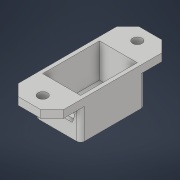
# Autodesk Inventor part: Caixa mlx
Saved by Autodesk Inventor 2021 (Build 250183000, 183)
## iProperties
Created: 2022-03-10
Part Number: Caixa mlx
Material: Genérico
Document SubType Name: Modeling
Designer: Hanter
Density: 1 g/cm^3
Appearance: Padrão
Author: Hanter
Autodesk Inventor part; units mm, degrees
ref_plane "YZ Plane" through (0, 0, 0) normal (1, 0, 0) x (0, 1, 0)
ref_plane "XZ Plane" through (0, 0, 0) normal (0, 1, 0) x (-1, 0, 0)
ref_plane "XY Plane" through (0, 0, 0) normal (0, 0, 1) x (1, 0, 0)
sketch "Esboço1" plane through (0, 0, 0) normal (0, 1, 0) x (-1, 0, 0)
  line L0 (-12, 17) -> (12, 17)
  line L1 (12, 17) -> (12, -17)
  line L2 (12, -17) -> (-12, -17)
  line L3 (-12, -17) -> (-12, 17)
  line L4 (-12, 17) -> (12, -17) construction
  line L5 (12, 17) -> (-12, -17) construction
  point P0 (0, 0)
  dimension "d0" = 24
  dimension "d1" = 34
  constraints: 12 end point, 2 midpoint, 2 parallel, 1 horizontal, 1 perpendicular
  measures "d0" distance of L1.end L2.end
  measures "d1" distance of L0.end L1.end
extrude "Extrusão1" add sketch "Esboço1" along normal blind 20
shell "Casca1" thickness 2 removed faces 1 at (4, 20, 5.6667)
sketch "Esboço2" plane through (-10, 2, 15) normal (0, 1, 0) x (1, 0, 0)
  line L0 (16, 8) -> (4, 8)
  line L1 (4, 8) -> (4, 25)
  line L2 (4, 25) -> (16, 25)
  line L3 (16, 25) -> (16, 8)
  line L4 (16, 8) -> (4, 25) construction
  line L5 (4, 8) -> (16, 25) construction
  line L6 (0, 30) -> (20, 30) projected
  circle A0 centre (6.5, 22.5) radius 1.5
  circle A1 centre (13.5, 22.5) radius 1.5
  point P0 (10, 15)
  point P1 (10, 16.5)
  dimension "d5" = 12
  dimension "d6" = 17
  dimension "d7" = 5
  dimension "d8" = 3
  dimension "d9" = 2.5
  dimension "d10" = 2.5
  dimension "d11" = 3
  dimension "d12" = 2.5
  constraints: 12 end point, 2 centre point, 2 midpoint, 2 parallel, 1 horizontal, 1 perpendicular
  measures "d5" distance of L1.end L2.end
  measures "d6" distance of L0.end L1.end
  measures "d7" distance between parallel lines of L6 L2
  measures "d8" diameter of A0
  measures "d9" distance from line of L1 A0.centre
  measures "d10" distance from line of L2 A0.centre
  measures "d11" diameter of A1
  measures "d12" distance from line of L3 A1.centre
extrude "Extrusão2" cut sketch "Esboço2" against normal blind 30 contours A0 | A1
sketch "Esboço3" plane through (0, 20, 0) normal (0, 1, 0) x (1, 0, 0)
  line L0 (12, 17) -> (-12, 17) projected
  line L1 (-12, 17) -> (12, 17)
  line L2 (12, 17) -> (12, 32)
  line L3 (12, 32) -> (-12, 32)
  line L4 (-12, 32) -> (-12, 17)
  line L5 (12, -17) -> (-12, -17) projected
  line L6 (-12, -17) -> (12, -17)
  line L7 (12, -17) -> (12, -32)
  line L8 (12, -32) -> (-12, -32)
  line L9 (-12, -32) -> (-12, -17)
  point P0 (0, 0)
  dimension "d15" = 24
  dimension "d16" = 15
  dimension "d17" = 15
  constraints: 16 end point, 4 parallel, 2 horizontal, 2 perpendicular, 1 point on line
  measures "d15" distance of L3.end L2.end
  measures "d16" distance of L2.end L1.end
  measures "d17" distance of L6.end L7.end
extrude "Extrusão3" add sketch "Esboço3" against normal blind 4
sketch "Esboço4" plane through (0, 16, 0) normal (0, -1, 0) x (1, 0, 0)
  circle A0 centre (0, 25) radius 2.5
  circle A1 centre (0, -25) radius 2.5
  line L0 (12, 17) -> (-12, 17) projected
  line L1 (-12, -17) -> (12, -17) projected
  point P0 (0, 0)
  dimension "d20" = 5
  dimension "d21" = 5
  dimension "d22" = 8
  dimension "d23" = 8
  dimension "d52" = 50
  constraints: 2 centre point
  measures "d20" diameter of A0
  measures "d21" diameter of A1
  measures "d22" distance from line of L0 A0.centre
  measures "d23" distance from line of L1 A1.centre
  measures "d52" distance of A1.centre A0.centre
extrude "Extrusão4" cut sketch "Esboço4" against normal blind 4
chamfer "Chanfro1" distance 6 angle 45 2 edges at (-12, 18, 32) (12, 18, 32)
chamfer "Chanfro2" distance 6 angle 45 2 edges at (12, 18, -32) (-12, 18, -32)
sketch "Esboço5" plane through (-10, 2, 15) normal (0, 1, 0) x (1, 0, 0)
  circle A0 centre (13.5, 22.5) radius 1.5 projected
  arc A1 (11.65, 22.5) -> (15.35, 22.5) centre (13.5, 22.5) ccw
  circle A2 centre (13.5, 22.5) radius 1.5
  circle A3 centre (6.5, 22.5) radius 1.5 projected
  circle A4 centre (6.5, 22.5) radius 1.5
  arc A5 (4.65, 22.5) -> (8.35, 22.5) centre (6.5, 22.5) ccw
  arc A6 (16.5, 22.5) -> (10.5, 22.5) centre (13.5, 22.5) ccw
  arc A7 (9.5, 22.5) -> (3.5, 22.5) centre (6.5, 22.5) ccw
  line L0 (15.35, 22.5) -> (16.5, 22.5)
  line L1 (11.65, 22.5) -> (10.5, 22.5)
  line L2 (8.35, 22.5) -> (9.5, 22.5)
  line L3 (3.5, 22.5) -> (4.65, 22.5)
  point P0 (10, 15)
  dimension "d32" = 3.7
  dimension "d33" = 3.7
  dimension "d34" = 6
  dimension "d35" = 6
  constraints: 8 end point, 8 point on circle, 6 centre point, 6 coincident, 6 point on line, 1 horizontal
  measures "d32" diameter of A1
  measures "d33" diameter of A5
  measures "d34" diameter of A6
  measures "d35" diameter of A7
extrude "Extrusão5" add sketch "Esboço5" along normal blind 0.8
sketch "Esboço6" plane through (-10, 2, 15) normal (0, 1, 0) x (1, 0, 0)
  circle A0 centre (10, 17) radius 4.1
  line L0 (16, 8) -> (4, 8)
  line L1 (4, 8) -> (4, 25)
  line L2 (4, 25) -> (16, 25)
  line L3 (16, 25) -> (16, 8)
  line L4 (16, 8) -> (4, 25) construction
  line L5 (4, 8) -> (16, 25) construction
  line L6 (0, 30) -> (20, 30) projected
  point P0 (10, 15)
  point P1 (10, 16.5)
  dimension "d38" = 8.2
  dimension "d39" = 12
  dimension "d40" = 17
  dimension "d41" = 5
  dimension "d42" = 9
  constraints: 12 end point, 2 midpoint, 2 parallel, 1 centre point, 1 horizontal, 1 perpendicular
  measures "d38" diameter of A0
  measures "d39" distance of L1.end L2.end
  measures "d40" distance of L0.end L1.end
  measures "d41" distance between parallel lines of L6 L2
  measures "d42" distance from line of L0 A0.centre
extrude "Extrusão6" cut sketch "Esboço6" against normal blind 2 contours A0
sketch "Esboço7" plane through (-12, 0, 17) normal (0, 0, 1) x (1, 0, 0)
  line L0 (4.5, 7.5) -> (19.5, 7.5)
  line L1 (19.5, 14.5) -> (4.5, 14.5)
  line L2 (4.5, 7.5) -> (19.5, 14.5) construction
  line L3 (19.5, 7.5) -> (4.5, 14.5) construction
  arc A0 (4.5, 14.5) -> (4.5, 7.5) centre (9.3734, 11) ccw
  arc A1 (19.5, 7.5) -> (19.5, 14.5) centre (14.6266, 11) ccw
  line L4 (24, 0) -> (0, 0) projected
  point P0 (12, 0)
  point P1 (12, 11)
  dimension "d47" = 6
  dimension "d48" = 6
  dimension "d51" = 15
  dimension "d56" = 7.5
  constraints: 8 end point, 4 point on circle, 2 centre point, 2 midpoint, 1 horizontal, 1 parallel
  measures "d47" radius of A0
  measures "d48" radius of A1
  measures "d51" distance of L1.start L1.end
  measures "d56" distance between parallel lines of L4 L0
extrude "Extrusão7" cut sketch "Esboço7" against normal blind 2
fillet "Fillet3" radius 2 4 edges at (12, 8, 17) (12, 8, -17) (-12, 8, -17) (-12, 8, 17)
